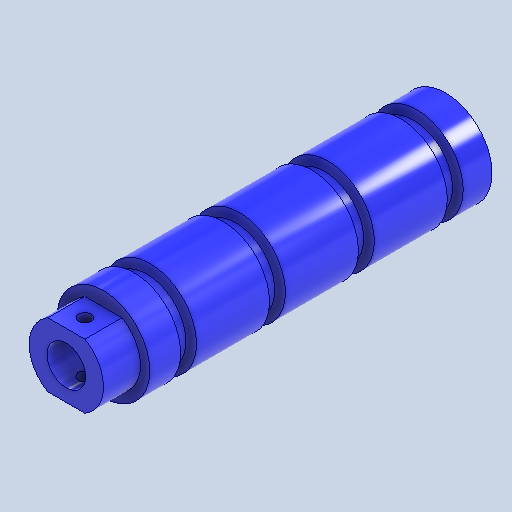
# Autodesk Inventor part: ball_loading_v1_3DP_P_B
Saved by Autodesk Inventor 2025.1 (Build 291241000, 241)
## iProperties
Created: 2024-11-12
Part Number: ball_loading_v1_3DP_P_B
Material: ABS プラスチック
Document SubType Name: Modeling
Designer: haruy
Density: 1.06 g/cm^3
Appearance: 青 - 壁塗料 - 光沢
Author: haruy
Autodesk Inventor part; units mm, degrees
ref_plane "YZ Plane" through (0, 0, 0) normal (1, 0, 0) x (0, 1, 0)
ref_plane "XY Plane" through (0, 0, 0) normal (0, 0, 1) x (1, 0, 0)
sketch "スケッチ1" plane through (0, 0, 0) normal (1, 0, 0) x (0, 1, 0)
  line L0 (0, -9.065995) -> (0, 0.934005)
  line L1 (0, 0) -> (12.5, 0)
  line L2 (12.5, 0) -> (12.5, -2.385786)
  line L3 (12.5, -2.385786) -> (10.5, -3.060246)
  line L4 (10.5, -3.060246) -> (10.5, -5.803392)
  line L5 (10.5, -5.803392) -> (12.5, -6.680209)
  line L6 (12.5, -6.680209) -> (12.5, -9.065995)
  line L7 (12.5, -9.065995) -> (0, -9.065995)
  line L8 (0, -9.065995) -> (0, 0)
  line L9 (10.5, -4.431819) -> (0, -4.532998)
  line L10 (10.5, -27.060246) -> (10.5, -29.803392)
  line L11 (12.5, -30.680209) -> (12.5, -33.065995)
  line L12 (10.5, -29.803392) -> (12.5, -30.680209)
  line L13 (12.5, -26.385786) -> (10.5, -27.060246)
  line L14 (12.5, -24) -> (12.5, -26.385786)
  line L15 (0, -24) -> (12.5, -24)
  line L16 (12.5, -33.065995) -> (0, -33.065995)
  line L17 (10.5, -28.431819) -> (0, -28.532998)
  line L18 (0, -33.065995) -> (0, -23.065995)
  line L19 (0, -33.065995) -> (0, -24)
  line L20 (10.5, -51.060246) -> (10.5, -53.803392)
  line L21 (12.5, -54.680209) -> (12.5, -57.065995)
  line L22 (10.5, -53.803392) -> (12.5, -54.680209)
  line L23 (12.5, -50.385786) -> (10.5, -51.060246)
  line L24 (12.5, -48) -> (12.5, -50.385786)
  line L25 (0, -48) -> (12.5, -48)
  line L26 (12.5, -57.065995) -> (0, -57.065995)
  line L27 (10.5, -52.431819) -> (0, -52.532998)
  line L28 (0, -57.065995) -> (0, -47.065995)
  line L29 (0, -57.065995) -> (0, -48)
  line L30 (10.5, -75.060246) -> (10.5, -77.803392)
  line L31 (12.5, -78.680209) -> (12.5, -81.065995)
  line L32 (10.5, -77.803392) -> (12.5, -78.680209)
  line L33 (12.5, -74.385786) -> (10.5, -75.060246)
  line L34 (12.5, -72) -> (12.5, -74.385786)
  line L35 (0, -72) -> (12.5, -72)
  line L36 (12.5, -81.065995) -> (0, -81.065995)
  line L37 (10.5, -76.431819) -> (0, -76.532998)
  line L38 (0, -81.065995) -> (0, -71.065995)
  line L39 (0, -81.065995) -> (0, -72)
  line L40 (0, -81.065995) -> (12.5, -81.065995)
  line L41 (12.5, -81.065995) -> (12.5, -86.473236)
  line L42 (12.5, -86.473236) -> (0, -86.473236)
  line L43 (0, -86.473236) -> (0, -81.065995)
  line L44 (12.5, -72) -> (12.5, -57.065995)
  line L45 (12.5, -48) -> (12.5, -33.065995)
  line L46 (12.5, -24) -> (12.5, -9.065995)
  line L47 (0, 0) -> (12.5, 0)
  line L48 (12.5, 0) -> (12.5, 5.934005)
  line L49 (12.5, 5.934005) -> (0, 5.934005)
  line L50 (0, 5.934005) -> (0, 0)
  line L51 (0, 5.934005) -> (10, 5.934005)
  line L52 (10, 5.934005) -> (10, 15.934005)
  line L53 (10, 15.934005) -> (0, 15.934005)
  line L54 (0, 15.934005) -> (0, 5.934005)
  line L55 (0, 15.934005) -> (0, -71.065995)
  circle A0 centre (12.5, -4.496449) radius 2
  point P0 (0, 0)
  point P1 (6.25, -86.473236)
  point P2 (0, -4.065995)
  point P3 (0, 0)
  point P4 (0, -23.065995)
  point P5 (0, -33.065995)
  point P6 (0, -47.065995)
  point P7 (0, -57.065995)
  point P8 (10, 5.934005)
  dimension "d1" = 2.74315
  dimension "d2" = 12.5
  dimension "d7" = 12.5
  dimension "d8" = 10
  dimension "d9" = 2.38579
  dimension "d10" = 2.38579
  dimension "d11" = 90
  dimension "d12" = 90
  dimension "d13" = 90
  dimension "d14" = 0
  dimension "d17" = 24
  dimension "d22" = 10
  dimension "d23" = 0
  dimension "d24" = 0
  dimension "d25" = 10
  dimension "d26" = 10
  dimension "d27" = 10
  dimension "d44" = 4
  dimension "d45" = 10.5
  dimension "d46" = 108.636
  constraints: 112 end point, 9 parallel, 4 midpoint, 4 perpendicular, 3 collinear, 3 horizontal, 3 tangent, 2 vertical, 1 centre point, 65 other
  measures "d1" distance of L3.end L4.end
  measures "d2" distance of L1.start L1.end
  measures "d7" distance of L6.end L7.end
  measures "d8" distance of L0.start L0.end
  measures "d9" distance of L5.end L6.end
  measures "d10" distance of L1.end L2.end
  measures "d14" distance from line of point (0, 0) L8
  measures "d17" distance of L3.end L10.start
  measures "d22" distance from line of point (6.25, -86.473) L37
  measures "d23" distance between parallel lines of L31 L41
  measures "d24" distance between parallel lines of L2 L48
  measures "d25" distance from line of L49 point (0, -4.066)
  measures "d26" distance of L53.end L52.end
  measures "d27" distance of L52.end L51.end
  measures "d44" diameter of A0
  measures "d45" distance between parallel lines of L0 L4
sketch "スケッチ1 outline for 回転1" plane through (0, 0, 0) normal (1, 0, 0) x (0, 1, 0)
  line L0 (10, 15.934005) -> (0, 15.934005)
  line L1 (10, 5.934005) -> (10, 15.934005)
  line L2 (12.5, 5.934005) -> (10, 5.934005)
  line L3 (12.5, 0) -> (12.5, 5.934005)
  line L4 (12.5, -2.385786) -> (12.5, 0)
  line L5 (10.5, -3.060246) -> (12.5, -2.385786)
  line L6 (10.5, -5.803392) -> (10.5, -3.060246)
  line L7 (12.5, -6.680209) -> (10.5, -5.803392)
  line L8 (12.5, -9.065995) -> (12.5, -6.680209)
  line L9 (12.5, -24) -> (12.5, -9.065995)
  line L10 (12.5, -26.385786) -> (12.5, -24)
  line L11 (10.5, -27.060246) -> (12.5, -26.385786)
  line L12 (10.5, -29.803392) -> (10.5, -27.060246)
  line L13 (12.5, -30.680209) -> (10.5, -29.803392)
  line L14 (12.5, -33.065995) -> (12.5, -30.680209)
  line L15 (12.5, -48) -> (12.5, -33.065995)
  line L16 (12.5, -50.385786) -> (12.5, -48)
  line L17 (10.5, -51.060246) -> (12.5, -50.385786)
  line L18 (10.5, -53.803392) -> (10.5, -51.060246)
  line L19 (12.5, -54.680209) -> (10.5, -53.803392)
  line L20 (12.5, -57.065995) -> (12.5, -54.680209)
  line L21 (12.5, -72) -> (12.5, -57.065995)
  line L22 (12.5, -74.385786) -> (12.5, -72)
  line L23 (10.5, -75.060246) -> (12.5, -74.385786)
  line L24 (10.5, -77.803392) -> (10.5, -75.060246)
  line L25 (12.5, -78.680209) -> (10.5, -77.803392)
  line L26 (12.5, -81.065995) -> (12.5, -78.680209)
  line L27 (12.5, -86.473236) -> (12.5, -81.065995)
  line L28 (0, -86.473236) -> (12.5, -86.473236)
  line L29 (0, -81.065995) -> (0, -86.473236)
  line L30 (0, -71.065995) -> (0, -81.065995)
  line L31 (0, -57.065995) -> (0, -71.065995)
  line L32 (0, -47.065995) -> (0, -57.065995)
  line L33 (0, -33.065995) -> (0, -47.065995)
  line L34 (0, -23.065995) -> (0, -33.065995)
  line L35 (0, -9.065995) -> (0, -23.065995)
  line L36 (0, 0) -> (0, -9.065995)
  line L37 (0, 5.934005) -> (0, 0)
  line L38 (0, 15.934005) -> (0, 5.934005)
revolve "回転1" add sketch "スケッチ1 outline for 回転1" angle 360 about axis through (0, 0, 15.934005) along (0, 0, -1)
sketch "スケッチ2" plane through (0, 0, -86.473236) normal (0, 0, -1) x (-1, 0, 0)
  circle A0 centre (0, 0) radius 5.2
  point P0 (0, 0)
  dimension "d29" = 10.4
  constraints: 1 centre point, 1 coincident
  measures "d29" diameter of A0
extrude "押し出し1" cut sketch "スケッチ2" against normal through all
ref_plane "作業平面1" through (0, -10, 10.934005) normal (0, 1, 0) x (-1, 0, 0)
sketch "スケッチ3" plane through (0, -10, 10.934005) normal (0, 1, 0) x (-1, 0, 0)
  line L0 (-10, 5) -> (10, 5) projected
  point P0 (0, -10.934005)
  point P1 (0, 0)
  dimension "d32" = 5
  measures "d32" distance from line of point (0, 0) L0
hole "穴1" at (0, -10, 10.934005) direction (0, 1, 0) diameter 3.4 end through all
sketch "スケッチ4" plane through (0, 0, 15.934005) normal (0, 0, 1) x (1, 0, 0)
  circle A0 centre (0, 0) radius 10
  line L0 (5, -8.660254) -> (-5, -8.660254)
  line L1 (10, 0) -> (-10, 0)
  line L2 (5, 8.660254) -> (-5, 8.660254)
  point P0 (0, 0)
  dimension "d40" = 10
  dimension "d41" = 20
  constraints: 6 end point, 4 point on circle, 2 symmetric about line, 1 centre point, 1 coincident, 1 horizontal
  measures "d40" distance of L0.start L0.end
  measures "d41" diameter of A0
extrude "押し出し2" cut sketch "スケッチ4" against normal blind 10 contours L2 A0 | A0 L0
